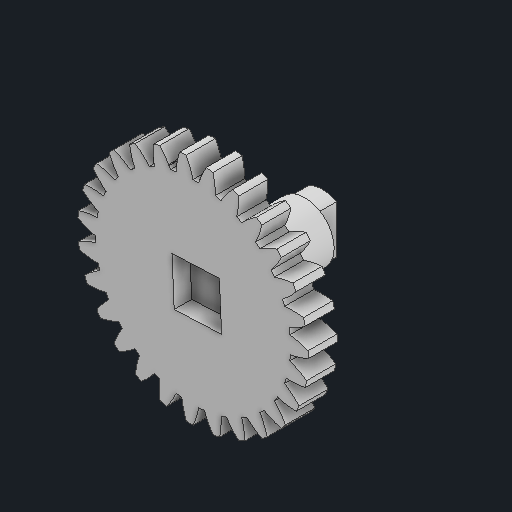
# Autodesk Inventor part: central axel
Saved by Autodesk Inventor 2026 (Build 300175050, 175E)
## iProperties
Created: 2026-03-26
Part Number: central axel
Material: Generic
Document SubType Name: Modeling
Designer: sniel
Density: 1 g/cm^3
Appearance: Default
Author: sniel
Autodesk Inventor part; units mm, degrees
ref_plane "YZ Plane" through (0, 0, 0) normal (1, 0, 0) x (0, 1, 0)
ref_plane "XZ Plane" through (0, 0, 0) normal (0, 1, 0) x (-1, 0, 0)
ref_plane "XY Plane" through (0, 0, 0) normal (0, 0, 1) x (1, 0, 0)
sketch "Sketch1" plane through (0, 0, 0) normal (0, 0, 1) x (1, 0, 0)
  arc A0 (-2.5, -4.3301) -> (2.5, -4.3301) centre (0, 0) ccw
  line L0 (2.5, 4.3301) -> (2.5, -4.3301)
  arc A1 (2.5, 4.3301) -> (-2.5, 4.3301) centre (0, 0) ccw
  line L1 (-2.5, -4.3301) -> (-2.5, 4.3301)
  line L2 (0, -5) -> (0, -4.75)
  circle A2 centre (0, 0) radius 4.75
  line L3 (-2.5, 0) -> (-2.4, 0)
  line L4 (2.5, 0) -> (2.4, 0)
  line L5 (-2.4, 0) -> (-2.4, -4.3863)
  line L6 (2.4, 0) -> (2.4, -4.3863)
  line L7 (2.4, 0) -> (2.4, 4.3863)
  line L8 (-2.4, 0) -> (-2.4, 4.3863)
  point P0 (0, 0)
  point P1 (-2.4, 4.0991)
  point P2 (-2.4, -4.0991)
  point P3 (2.4, -4.0991)
  point P4 (2.4, 4.0991)
  dimension "d0" = 0.25
  dimension "d1" = 0.1
  dimension "d2" = 0.1
  constraints: 18 end point, 9 point on circle, 4 vertical, 2 centre point, 2 horizontal, 2 midpoint, 1 coincident, 3 other
  measures "d0" distance of L2.start L2.end
  measures "d1" distance of L3.start L3.end
  measures "d2" distance of L4.start L4.end
extrude "Extrusion1" add sketch "Sketch1" along normal blind 3 contours L5 L8 A2 L7 L6
ref_plane "Work Plane1" through (-110.4204, -110.4204, 21.5411) normal (0, 0, -1) x (-0.0507737, 0.9987102, 0)
sketch "Sketch2" plane through (0, 0, 3) normal (0, 0, 1) x (1, 0, 0)
  circle A0 centre (0, 0) radius 5
  dimension "d5" = 10
  constraints: 1 centre point, 1 coincident
  measures "d5" diameter of A0
extrude "Extrusion2" add sketch "Sketch2" along normal up to surface (18.5411 mm away)
sketch "Sketch3" plane through (0, 0, 21.5411) normal (0, 0, 1) x (1, 0, 0)
  arc A0 (-4.8284, 16.7732) -> (-6.3222, 18.8577) centre (-16.1161, 10.2619) ccw
  arc A1 (-6.3222, 18.8577) -> (-7.4127, 18.4955) centre (-0.6419, -0.0624) ccw
  arc A2 (-7.4127, 18.4955) -> (-7.264, 15.2567) centre (5.5779, 17.4691) ccw
  arc A3 (-7.264, 15.2567) -> (-8.1435, 14.8457) centre (-0.6419, -0.0624) ccw
  arc A4 (-8.1435, 14.8457) -> (-10.5324, 17.0378) centre (-18.0799, 6.415) ccw
  arc A5 (-10.5324, 17.0378) -> (-11.5099, 16.4338) centre (-0.6419, -0.0624) ccw
  arc A6 (-11.5099, 16.4338) -> (-10.6183, 13.3166) centre (1.3672, 18.4309) ccw
  arc A7 (-10.6183, 13.3166) -> (-11.3793, 12.7139) centre (-0.6419, -0.0624) ccw
  arc A8 (-11.3793, 12.7139) -> (-14.2093, 14.296) centre (-19.1036, 2.2189) ccw
  arc A9 (-14.2093, 14.296) -> (-15.0212, 13.4828) centre (-0.6419, -0.0624) ccw
  arc A10 (-15.0212, 13.4828) -> (-13.4348, 10.6552) centre (-2.9518, 18.3958) ccw
  arc A11 (-13.4348, 10.6552) -> (-14.0363, 9.8933) centre (-0.6419, -0.0624) ccw
  arc A12 (-14.0363, 9.8933) -> (-17.1549, 10.7801) centre (-19.1321, -2.1002) ccw
  arc A13 (-17.1549, 10.7801) -> (-17.7574, 9.8016) centre (-0.6419, -0.0624) ccw
  arc A14 (-17.7574, 9.8016) -> (-15.5616, 7.4161) centre (-7.1463, 17.3655) ccw
  arc A15 (-15.5616, 7.4161) -> (-15.9712, 6.5359) centre (-0.6419, -0.0624) ccw
  arc A16 (-15.9712, 6.5359) -> (-19.2102, 6.6796) centre (-18.1638, -6.3094) ccw
  arc A17 (-19.2102, 6.6796) -> (-19.5708, 5.5886) centre (-0.6419, -0.0624) ccw
  arc A18 (-19.5708, 5.5886) -> (-16.8841, 3.7738) centre (-10.9901, 15.3958) ccw
  arc A19 (-16.8841, 3.7738) -> (-17.0797, 2.8229) centre (-0.6419, -0.0624) ccw
  arc A20 (-17.0797, 2.8229) -> (-20.2645, 2.2158) centre (-16.2508, -10.1818) ccw
  arc A21 (-20.2645, 2.2158) -> (-20.3638, 1.0709) centre (-0.6419, -0.0624) ccw
  arc A22 (-20.3638, 1.0709) -> (-17.331, -0.0753) centre (-14.2761, 12.5926) ccw
  arc A23 (-17.331, -0.0753) -> (-17.302, -1.0457) centre (-0.6419, -0.0624) ccw
  arc A24 (-17.302, -1.0457) -> (-20.261, -2.3709) centre (-13.4964, -13.5087) ccw
  arc A25 (-20.261, -2.3709) -> (-20.0936, -3.5078) centre (-0.6419, -0.0624) ccw
  arc A26 (-20.0936, -3.5078) -> (-16.8782, -3.9237) centre (-16.827, 9.1072) ccw
  arc A27 (-16.8782, -3.9237) -> (-16.6262, -4.8613) centre (-0.6419, -0.0624) ccw
  arc A28 (-16.6262, -4.8613) -> (-19.1998, -6.8332) centre (-10.049, -16.1107) ccw
  arc A29 (-19.1998, -6.8332) -> (-18.7747, -7.9008) centre (-0.6419, -0.0624) ccw
  arc A30 (-18.7747, -7.9008) -> (-15.55, -7.564) centre (-18.5054, 5.1275) ccw
  arc A31 (-15.55, -7.564) -> (-15.0886, -8.4181) centre (-0.6419, -0.0624) ccw
  arc A32 (-15.0886, -8.4181) -> (-17.1381, -10.9304) centre (-6.0944, -17.8475) ccw
  arc A33 (-17.1381, -10.9304) -> (-16.4783, -11.8712) centre (-0.6419, -0.0624) ccw
  arc A34 (-16.4783, -11.8712) -> (-13.4182, -10.7998) centre (-19.2208, 0.868) ccw
  arc A35 (-13.4182, -10.7998) -> (-12.7722, -11.5246) centre (-0.6419, -0.0624) ccw
  arc A36 (-12.7722, -11.5246) -> (-14.1871, -14.4418) centre (-1.8459, -18.6256) ccw
  arc A37 (-14.1871, -14.4418) -> (-13.3281, -15.205) centre (-0.6419, -0.0624) ccw
  arc A38 (-13.3281, -15.205) -> (-10.5976, -13.4568) centre (-18.9346, -3.4416) ccw
  arc A39 (-10.5976, -13.4568) -> (-9.8019, -14.013) centre (-0.6419, -0.0624) ccw
  arc A40 (-9.8019, -14.013) -> (-10.5059, -17.1779) centre (2.4675, -18.4029) ccw
  arc A41 (-10.5059, -17.1779) -> (-9.494, -17.7225) centre (-0.6419, -0.0624) ccw
  arc A42 (-9.494, -17.7225) -> (-7.2402, -15.3917) centre (-17.6622, -7.5691) ccw
  arc A43 (-7.2402, -15.3917) -> (-6.3378, -15.7494) centre (-0.6419, -0.0624) ccw
  arc A44 (-6.3378, -15.7494) -> (-6.2929, -18.9913) centre (6.6133, -17.1914) ccw
  arc A45 (-6.2929, -18.9913) -> (-5.1827, -19.2879) centre (-0.6419, -0.0624) ccw
  arc A46 (-5.1827, -19.2879) -> (-3.5272, -16.5002) centre (-15.4722, -11.2919) ccw
  arc A47 (-3.5272, -16.5002) -> (-2.5666, -16.6401) centre (-0.6419, -0.0624) ccw
  arc A48 (-2.5666, -16.6401) -> (-1.7752, -19.7843) centre (10.3679, -15.0565) ccw
  arc A49 (-1.7752, -19.7843) -> (-0.6266, -19.8168) centre (-0.6419, -0.0624) ccw
  arc A50 (-0.6266, -19.8168) -> (0.3414, -16.7225) centre (-12.4828, -14.4093) ccw
  arc A51 (0.3414, -16.7225) -> (1.3084, -16.6371) centre (-0.6419, -0.0624) ccw
  arc A52 (1.3084, -16.6371) -> (2.8035, -19.5141) centre (13.5291, -12.1133) ccw
  arc A53 (2.8035, -19.5141) -> (3.9287, -19.2808) centre (-0.6419, -0.0624) ccw
  arc A54 (3.9287, -19.2808) -> (4.157, -16.0467) centre (-8.8549, -16.7533) ccw
  arc A55 (4.157, -16.0467) -> (5.0782, -15.7406) centre (-0.6419, -0.0624) ccw
  arc A56 (5.0782, -15.7406) -> (7.1965, -18.1952) centre (15.9262, -8.5204) ccw
  arc A57 (7.1965, -18.1952) -> (8.2375, -17.7087) centre (-0.6419, -0.0624) ccw
  arc A58 (8.2375, -17.7087) -> (7.7138, -14.5091) centre (-4.7844, -18.1975) ccw
  arc A59 (7.7138, -14.5091) -> (8.5397, -13.9988) centre (-0.6419, -0.0624) ccw
  arc A60 (8.5397, -13.9988) -> (11.1669, -15.8988) centre (17.4302, -4.4716) ccw
  arc A61 (11.1669, -15.8988) -> (12.0677, -15.1853) centre (-0.6419, -0.0624) ccw
  arc A62 (12.0677, -15.1853) -> (10.8202, -12.1927) centre (-0.4905, -18.664) ccw
  arc A63 (10.8202, -12.1927) -> (11.5062, -11.5058) centre (-0.6419, -0.0624) ccw
  arc A64 (11.5062, -11.5058) -> (14.5007, -12.7486) centre (17.9599, -0.185) ccw
  arc A65 (14.5007, -12.7486) -> (15.2127, -11.8467) centre (-0.6419, -0.0624) ccw
  arc A66 (15.2127, -11.8467) -> (13.3087, -9.2224) centre (3.7952, -18.1276) ccw
  arc A67 (13.3087, -9.2224) -> (13.8177, -8.3958) centre (-0.6419, -0.0624) ccw
  arc A68 (13.8177, -8.3958) -> (17.0182, -8.9145) centre (17.4867, 4.1081) ccw
  arc A69 (17.0182, -8.9145) -> (17.503, -7.8727) centre (-0.6419, -0.0624) ccw
  arc A70 (17.503, -7.8727) -> (15.0451, -5.7583) centre (7.8418, -16.6174) ccw
  arc A71 (15.0451, -5.7583) -> (15.3498, -4.8365) centre (-0.6419, -0.0624) ccw
  arc A72 (15.3498, -4.8365) -> (18.5836, -4.6032) centre (16.0363, 8.1765) ccw
  arc A73 (18.5836, -4.6032) -> (18.8151, -3.4777) centre (-0.6419, -0.0624) ccw
  arc A74 (18.8151, -3.4777) -> (15.9358, -1.9871) centre (11.4309, -14.2147) ccw
  arc A75 (15.9358, -1.9871) -> (16.0197, -1.0199) centre (-0.6419, -0.0624) ccw
  arc A76 (16.0197, -1.0199) -> (19.1125, -0.0471) centre (13.6867, 11.8006) ccw
  arc A77 (19.1125, -0.0471) -> (19.0782, 1.1015) centre (-0.6419, -0.0624) ccw
  arc A78 (19.0782, 1.1015) -> (15.9328, 1.8879) centre (14.3693, -11.049) ccw
  arc A79 (15.9328, 1.8879) -> (15.7914, 2.8483) centre (-0.6419, -0.0624) ccw
  arc A80 (15.7914, 2.8483) -> (18.5765, 4.5082) centre (10.5647, 14.7853) ccw
  arc A81 (18.5765, 4.5082) -> (18.2783, 5.6179) centre (-0.6419, -0.0624) ccw
  arc A82 (18.2783, 5.6179) -> (15.0363, 5.6577) centre (16.4983, -7.2911) ccw
  arc A83 (15.0363, 5.6577) -> (14.6772, 6.5597) centre (-0.6419, -0.0624) ccw
  arc A84 (14.6772, 6.5597) -> (17.0044, 8.817) centre (6.8385, 16.9695) ccw
  arc A85 (17.0044, 8.817) -> (16.4583, 9.8281) centre (-0.6419, -0.0624) ccw
  arc A86 (16.4583, 9.8281) -> (13.2945, 9.1192) centre (17.7033, -3.1434) ccw
  arc A87 (13.2945, 9.1192) -> (12.7371, 9.914) centre (-0.6419, -0.0624) ccw
  arc A88 (12.7371, 9.914) -> (14.481, 12.6472) centre (2.709, 18.2355) ccw
  arc A89 (14.481, 12.6472) -> (13.7165, 13.505) centre (-0.6419, -0.0624) ccw
  arc A90 (13.7165, 13.505) -> (10.8014, 12.0857) centre (17.9194, 1.1703) ccw
  arc A91 (10.8014, 12.0857) -> (10.0757, 12.7305) centre (-0.6419, -0.0624) ccw
  arc A92 (10.0757, 12.7305) -> (11.1424, 15.7922) centre (-1.6011, 18.515) ccw
  arc A93 (11.1424, 15.7922) -> (10.2006, 16.4506) centre (-0.6419, -0.0624) ccw
  arc A94 (10.2006, 16.4506) -> (7.6915, 14.3972) centre (17.1348, 5.4176) ccw
  arc A95 (7.6915, 14.3972) -> (6.8366, 14.8573) centre (-0.6419, -0.0624) ccw
  arc A96 (6.8366, 14.8573) -> (7.1684, 18.0825) centre (-5.8595, 17.793) ccw
  arc A97 (7.1684, 18.0825) -> (6.1001, 18.5059) centre (-0.6419, -0.0624) ccw
  arc A98 (6.1001, 18.5059) -> (4.1322, 15.9293) centre (15.3918, 9.3695) ccw
  arc A99 (4.1322, 15.9293) -> (3.1943, 16.1798) centre (-0.6419, -0.0624) ccw
  arc A100 (3.1943, 16.1798) -> (2.7734, 19.3946) centre (-9.8366, 16.1085) ccw
  arc A101 (2.7734, 19.3946) -> (1.6363, 19.5602) centre (-0.6419, -0.0624) ccw
  arc A102 (1.6363, 19.5602) -> (0.5307, 17.2462) centre (12.7845, 12.8129) ccw
  arc A103 (0.5307, 17.2462) -> (0.5011, 17.1057) centre (20.0615, 13.0592) ccw
  arc A104 (0.5011, 17.1057) -> (0.4804, 17.1045) centre (5.7469, -72.441) ccw
  arc A105 (0.4804, 17.1045) -> (0.3156, 16.5992) centre (12.7845, 12.8129) ccw
  arc A106 (0.3156, 16.5992) -> (-0.6548, 16.6267) centre (-0.6419, -0.0624) ccw
  arc A107 (-0.6548, 16.6267) -> (-1.8058, 19.6577) centre (-13.318, 13.5522) ccw
  arc A108 (-1.8058, 19.6577) -> (-2.9504, 19.5567) centre (-0.6419, -0.0624) ccw
  arc A109 (-2.9504, 19.5567) -> (-3.5527, 16.3709) centre (9.4533, 15.5622) ccw
  arc A110 (-3.5527, 16.3709) -> (-4.5032, 16.1738) centre (-0.6419, -0.0624) ccw
  arc A111 (-4.5032, 16.1738) -> (-4.754, 16.6425) centre (-16.1161, 10.2619) ccw
  arc A112 (-4.754, 16.6425) -> (-4.7746, 16.64) centre (5.7469, -72.441) ccw
  arc A113 (-4.7746, 16.64) -> (-4.8284, 16.7732) centre (-23.3238, 9.2297) ccw
  point P0 (0, 0)
  constraints: 228 point on circle, 114 centre point
extrude "Extrusion3" add sketch "Sketch3" against normal blind 5
sketch "Sketch4" plane through (5.5779, 17.4691, 21.5411) normal (0, 0, 1) x (0.9989475, 0.0458672, 0)
  circle A0 centre (-6.3733, -17.1949) radius 5.75
  line L0 (-6.3733, -17.1949) -> (-2.3074, -21.2608)
  line L1 (-6.3733, -17.1949) -> (-0.6233, -17.1949) construction
  line L2 (-10.4392, -13.129) -> (-2.3074, -13.129)
  line L3 (-2.3074, -13.129) -> (-2.3074, -21.2608)
  line L4 (-2.3074, -21.2608) -> (-10.4392, -21.2608)
  line L5 (-10.4392, -21.2608) -> (-10.4392, -13.129)
  line L6 (-10.4392, -13.129) -> (-2.3074, -21.2608) construction
  line L7 (-2.3074, -13.129) -> (-10.4392, -21.2608) construction
  arc A1 (-6.4028, -11.181) -> (-6.3438, -23.2088) centre (-6.3733, -17.1949) ccw projected
  point P0 (-6.3733, -17.1949)
  dimension "d10" = 11.5
  dimension "d11" = 45
  constraints: 16 end point, 2 horizontal, 2 midpoint, 2 parallel, 1 equal length, 1 perpendicular, 3 other
  measures "d11" angle of L0 L1
extrude "Extrusion4" cut sketch "Sketch4" against normal blind 3 contours L3 L4 L5 L2
body "Solid1"
